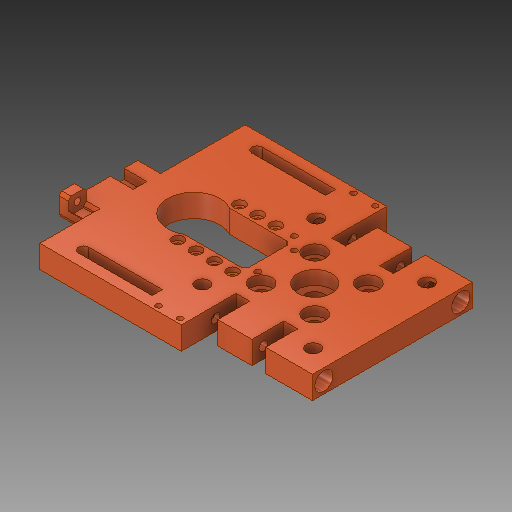
# Autodesk Inventor part: КВ33.044.901 - Щека каретки Z
Saved by Autodesk Inventor 2019 (Build 230136000, 136)
## iProperties
Created: 2019-08-08
Part Number: КВ33.044.901 - Щека каретки Z
Material: Пластик АБС
Document SubType Name: Modeling
Designer: user
Density: 1.06 g/cm^3
Appearance: Гладкий — светло-оранжевый
Mass: 66.4616 g
Surface Area: 302.013 cm^2
Volume: 62.6996 cm^3
Author: user
Autodesk Inventor part; units mm, degrees
(part 1 of 2)
ref_plane "YZ Plane" through (0, 0, 0) normal (1, 0, 0) x (0, 1, 0)
ref_plane "XZ Plane" through (0, 0, 0) normal (0, 1, 0) x (-1, 0, 0)
ref_plane "XY Plane" through (0, 0, 0) normal (0, 0, 1) x (1, 0, 0)
sketch "Эскиз4" plane through (0, 0, 0) normal (0, 1, 0) x (-1, 0, 0)
  circle A0 centre (-24.3, 25) radius 3
  circle A1 centre (24.3, 25) radius 3
  circle A2 centre (24.3, -25) radius 3
  circle A3 centre (-24.3, -25) radius 3
  line L0 (13.5, -21) -> (13.5, -35)
  line L1 (13.5, -35) -> (34, -35)
  line L2 (34, -35) -> (34, 35)
  line L3 (34, 35) -> (13.5, 35)
  line L4 (13.5, 35) -> (13.5, 21)
  line L5 (13.5, 21) -> (7.5, 21)
  line L6 (7.5, 21) -> (7.5, 35)
  line L7 (7.5, 35) -> (-7.5, 35)
  line L8 (-7.5, 35) -> (-7.5, 21)
  line L9 (-7.5, 21) -> (-13.5, 21)
  line L10 (-13.5, 21) -> (-13.5, 35)
  line L11 (-13.5, 35) -> (-34, 35)
  line L12 (-34, 35) -> (-34, -35)
  line L13 (-34, -35) -> (-13.5, -35)
  line L14 (-13.5, -35) -> (-13.5, -21)
  line L15 (-13.5, -21) -> (-7.5, -21)
  line L16 (-7.5, -21) -> (-7.5, -35)
  line L17 (-7.5, -35) -> (7.5, -35)
  line L18 (7.5, -35) -> (7.5, -21)
  line L19 (7.5, -21) -> (13.5, -21)
  circle A4 centre (0, 0) radius 7.5
  circle A5 centre (-11.75, 11.7501) radius 4.65
  circle A6 centre (-11.7501, -11.75) radius 4.65
  line L20 (26, 12) -> (16.3934, 12)
  line L21 (26, -12) -> (26, 12)
  line L22 (16.3933, -12) -> (26, -12)
  arc A7 (16, -9.8634) -> (16.3933, -12) centre (11.75, -11.7501) ccw
  line L23 (16, -9.8634) -> (16, 9.8629)
  arc A8 (16.3934, 12) -> (16, 9.8629) centre (11.7501, 11.75) ccw
  circle A9 centre (-11.75, 11.7501) radius 2.6
  circle A10 centre (-11.7501, -11.75) radius 2.6
  circle A11 centre (11.75, -11.7501) radius 2.6
  circle A12 centre (11.7501, 11.75) radius 2.6
  circle A13 centre (0, 0) radius 4.1
  circle A14 centre (11.7501, 11.75) radius 4.65
  circle A15 centre (11.75, -11.7501) radius 4.65
  constraints: 48 end point, 14 centre point, 4 point on circle, 2 coincident, 6 other
extrude "Выдавливание3" add sketch "Эскиз4" along normal blind 10 contours L19 L18 L17 L16 L15 L14 L13 L12 L11 L10 L9 L8 L7 L6 L5 L4 L3 L2 L1 L0 | A4 | A5 | A6 | L21 L22 A15 L23 A14 L20 | A14 A8 | A7 A15
sketch "Эскиз5" plane through (0, 10, 0) normal (0, 1, 0) x (1, 0, 0)
  circle A0 centre (-24.3, 25) radius 3
  circle A1 centre (24.3, 25) radius 3
  circle A2 centre (24.3, -25) radius 3
  circle A3 centre (-24.3, -25) radius 3
  line L0 (13.5, -21) -> (13.5, -35)
  line L1 (13.5, -35) -> (34, -35)
  line L2 (34, -35) -> (34, 35)
  line L3 (34, 35) -> (13.5, 35)
  line L4 (13.5, 35) -> (13.5, 21)
  line L5 (13.5, 21) -> (7.5, 21)
  line L6 (7.5, 21) -> (7.5, 35)
  line L7 (7.5, 35) -> (-7.5, 35)
  line L8 (-7.5, 35) -> (-7.5, 21)
  line L9 (-7.5, 21) -> (-13.5, 21)
  line L10 (-13.5, 21) -> (-13.5, 35)
  line L11 (-13.5, 35) -> (-34, 35)
  line L12 (-34, 35) -> (-34, -35)
  line L13 (-34, -35) -> (-13.5, -35)
  line L14 (-13.5, -35) -> (-13.5, -21)
  line L15 (-13.5, -21) -> (-7.5, -21)
  line L16 (-7.5, -21) -> (-7.5, -35)
  line L17 (-7.5, -35) -> (7.5, -35)
  line L18 (7.5, -35) -> (7.5, -21)
  line L19 (7.5, -21) -> (13.5, -21)
  circle A4 centre (0, 0) radius 7.5
  circle A5 centre (-11.75, 11.7501) radius 4.65
  circle A6 centre (-11.7501, -11.75) radius 4.65
  line L20 (26, 12) -> (16.3934, 12)
  line L21 (26, -12) -> (26, 12)
  line L22 (16.3933, -12) -> (26, -12)
  arc A7 (16, -9.8634) -> (16.3933, -12) centre (11.75, -11.7501) ccw
  line L23 (16, -9.8634) -> (16, 9.8629)
  arc A8 (16.3934, 12) -> (16, 9.8629) centre (11.7501, 11.75) ccw
  circle A9 centre (-11.75, 11.7501) radius 2.6
  circle A10 centre (-11.7501, -11.75) radius 2.6
  circle A11 centre (11.75, -11.7501) radius 2.6
  circle A12 centre (11.7501, 11.75) radius 2.6
  circle A13 centre (0, 0) radius 4.1
  circle A14 centre (11.75, -11.7501) radius 2.6 projected
  circle A15 centre (11.75, -11.7501) radius 4.65
  circle A16 centre (11.7501, 11.75) radius 4.65
  constraints: 48 end point, 16 centre point, 4 point on circle, 2 coincident, 2 concentric
extrude "Выдавливание4" cut sketch "Эскиз5" against normal blind 4 contours A5 | A6 | A16 A8 | A7 A15
sketch "Эскиз6" plane through (0, 10, 0) normal (0, 1, 0) x (1, 0, 0)
  circle A0 centre (-24.3, 25) radius 3
  circle A1 centre (24.3, 25) radius 3
  circle A2 centre (24.3, -25) radius 3
  circle A3 centre (-24.3, -25) radius 3
  line L0 (13.5, -21) -> (13.5, -35)
  line L1 (13.5, -35) -> (34, -35)
  line L2 (34, -35) -> (34, 35)
  line L3 (34, 35) -> (13.5, 35)
  line L4 (13.5, 35) -> (13.5, 21)
  line L5 (13.5, 21) -> (7.5, 21)
  line L6 (7.5, 21) -> (7.5, 35)
  line L7 (7.5, 35) -> (-7.5, 35)
  line L8 (-7.5, 35) -> (-7.5, 21)
  line L9 (-7.5, 21) -> (-13.5, 21)
  line L10 (-13.5, 21) -> (-13.5, 35)
  line L11 (-13.5, 35) -> (-34, 35)
  line L12 (-34, 35) -> (-34, -35)
  line L13 (-34, -35) -> (-13.5, -35)
  line L14 (-13.5, -35) -> (-13.5, -21)
  line L15 (-13.5, -21) -> (-7.5, -21)
  line L16 (-7.5, -21) -> (-7.5, -35)
  line L17 (-7.5, -35) -> (7.5, -35)
  line L18 (7.5, -35) -> (7.5, -21)
  line L19 (7.5, -21) -> (13.5, -21)
  circle A4 centre (0, 0) radius 7.5
  circle A5 centre (-11.75, 11.7501) radius 4.65
  circle A6 centre (-11.7501, -11.75) radius 4.65
  line L20 (26, 12) -> (16.3934, 12)
  line L21 (26, -12) -> (26, 12)
  line L22 (16.3933, -12) -> (26, -12)
  arc A7 (16, -9.8634) -> (16.3933, -12) centre (11.75, -11.7501) ccw
  line L23 (16, -9.8634) -> (16, 9.8629)
  arc A8 (16.3934, 12) -> (16, 9.8629) centre (11.7501, 11.75) ccw
  circle A9 centre (-11.75, 11.7501) radius 2.6
  circle A10 centre (-11.7501, -11.75) radius 2.6
  circle A11 centre (11.75, -11.7501) radius 2.6
  circle A12 centre (11.7501, 11.75) radius 2.6
  circle A13 centre (0, 0) radius 4.1
  constraints: 48 end point, 14 centre point, 4 point on circle
extrude "Выдавливание5" cut sketch "Эскиз6" against normal blind 6 contours A4
sketch "Эскиз7" plane through (34, 0, 35) normal (1, 0, 0) x (0, 0, -1)
  circle A0 centre (5, 5) radius 2
  circle A1 centre (5, 5) radius 4
  circle A2 centre (65, 5) radius 4
  circle A3 centre (5, 5) radius 4
  line L0 (0, 0) -> (70, 0)
  line L1 (70, 0) -> (70, 10)
  line L2 (0, 10) -> (70, 10)
  line L3 (0, 0) -> (0, 10)
  circle A4 centre (65, 5) radius 2
  circle A5 centre (65, 5) radius 4
  point P0 (35, 0)
  point P1 (35, 0)
  constraints: 8 end point, 6 centre point
extrude "Выдавливание6" cut sketch "Эскиз7" against normal blind 269 contours A0 | A4
sketch "Эскиз8" plane through (34, 0, 35) normal (1, 0, 0) x (0, 0, -1)
  circle A0 centre (5, 5) radius 2
  circle A1 centre (5, 5) radius 4
  circle A2 centre (65, 5) radius 4
  circle A3 centre (5, 5) radius 4
  line L0 (0, 0) -> (70, 0)
  line L1 (70, 0) -> (70, 10)
  line L2 (0, 10) -> (70, 10)
  line L3 (0, 0) -> (0, 10)
  circle A4 centre (65, 5) radius 2
  circle A5 centre (65, 5) radius 4
  point P0 (35, 0)
  point P1 (35, 0)
  constraints: 8 end point, 6 centre point
extrude "Выдавливание7" cut sketch "Эскиз8" against normal blind 15 contours A1 | A2
sketch "Эскиз9" plane through (-34, 0, -35) normal (-1, 0, 0) x (0, 0, 1)
  circle A0 centre (5, 5) radius 2
  circle A1 centre (5, 5) radius 4
  circle A2 centre (65, 5) radius 4
  circle A3 centre (5, 5) radius 4
  line L0 (0, 0) -> (70, 0)
  line L1 (70, 0) -> (70, 10)
  line L2 (0, 10) -> (70, 10)
  line L3 (0, 0) -> (0, 10)
  circle A4 centre (65, 5) radius 2
  circle A5 centre (65, 5) radius 4
  point P0 (35, 0)
  point P1 (35, 0)
  constraints: 8 end point, 6 centre point
extrude "Выдавливание8" cut sketch "Эскиз9" against normal blind 15 contours A1 | A2
sketch "Эскиз17" plane through (-34, 0, -35) normal (-1, 0, 0) x (0, 0, 1)
  line L0 (14, 10) -> (0, 10) projected
  line L1 (70, 0) -> (56, 0) projected
  line L2 (0, 10) -> (70, 10)
  line L3 (70, 10) -> (70, 0)
  line L4 (70, 0) -> (0, 0)
  line L5 (0, 0) -> (0, 10)
  point P0 (35, 0)
  constraints: 8 end point, 2 parallel, 1 horizontal, 1 perpendicular
extrude "Выдавливание14" add sketch "Эскиз17" along normal blind 33
sketch "Эскиз18" plane through (0, 0, 0) normal (0, -1, 0) x (1, 0, 0)
  line L0 (-35.2, -12.6) -> (-35.2, -14.9)
  line L1 (-35.2, -12.6) -> (-33.8, -12.6)
  line L2 (-33.8, -14.9) -> (-33.8, -12.6)
  line L3 (-27.2, -14.9) -> (-33.8, -14.9)
  line L4 (-27.2, -12.6) -> (-27.2, -14.9)
  circle A0 centre (-53, 0) radius 9.15
  circle A1 centre (-53, 0) radius 1.5
  circle A2 centre (-17, 8) radius 1.3
  circle A3 centre (-30.5, 13.5) radius 1.3
  circle A4 centre (-22.5, 13.5) radius 1.3
  circle A5 centre (-38.5, 13.5) radius 1.3
  circle A6 centre (-46.5, 13.5) radius 1.3
  circle A7 centre (-17, -8) radius 1.3
  circle A8 centre (-30.5, -13.5) radius 1.3
  circle A9 centre (-22.5, -13.5) radius 1.3
  circle A10 centre (-38.5, -13.5) radius 1.3
  circle A11 centre (-46.5, -13.5) radius 1.3
  line L5 (-64.0198, -0.1) -> (-63.4796, -0.1)
  line L6 (-64.0198, -7) -> (-64.0198, -0.1)
  arc A12 (-64.0198, -7) -> (-63.9686, -7.75) centre (-58.5, -7) ccw
  line L7 (-61.5, -7.75) -> (-63.9686, -7.75)
  arc A13 (-59.75, -9.5) -> (-61.5, -7.75) centre (-61.5, -9.5) ccw
  line L8 (-59.75, -10) -> (-59.75, -9.5)
  line L9 (-22.1937, -10) -> (-59.75, -10)
  arc A14 (-22.1937, -10) -> (-21.5055, -9.6078) centre (-22.1937, -9.2) ccw
  arc A15 (-21.5055, -9.6078) -> (-20.8922, -8.9945) centre (-20, -10.5) ccw
  arc A16 (-20.8922, -8.9945) -> (-20.5, -8.3063) centre (-21.3, -8.3063) ccw
  line L10 (-20.5, 8.3063) -> (-20.5, -8.3063)
  arc A17 (-20.5, 8.3063) -> (-20.8922, 8.9945) centre (-21.3, 8.3063) ccw
  arc A18 (-21.5055, 9.6078) -> (-20.8922, 8.9945) centre (-20, 10.5) ccw
  arc A19 (-20.8922, 8.9945) -> (-21.5055, 9.6078) centre (-20, 10.5) ccw
  line L11 (-59.75, -11.3229) -> (-59.75, -10)
  arc A20 (-59.75, -11.3229) -> (-58.5, -11.5) centre (-58.4989, -6.9922) ccw
  line L12 (-58.5, -11.5) -> (-51, -11.5)
  line L13 (-51, -12.6) -> (-51, -11.5)
  line L14 (-49.8, -12.6) -> (-51, -12.6)
  line L15 (-49.8, -14.9) -> (-49.8, -12.6)
  line L16 (-43.2, -14.9) -> (-49.8, -14.9)
  line L17 (-43.2, -12.6) -> (-43.2, -14.9)
  line L18 (-41.8, -12.6) -> (-43.2, -12.6)
  line L19 (-41.8, -14.9) -> (-41.8, -12.6)
  line L20 (-35.2, -14.9) -> (-41.8, -14.9)
  line L21 (-35.2, -12.6) -> (-35.2, -14.9)
  line L22 (-33.8, -12.6) -> (-35.2, -12.6)
  line L23 (-33.8, -14.9) -> (-33.8, -12.6)
  line L24 (-27.2, -14.9) -> (-33.8, -14.9)
  line L25 (-27.2, -12.6) -> (-27.2, -14.9)
  line L26 (-25.8, -12.6) -> (-27.2, -12.6)
  line L27 (-25.8, -14.9) -> (-25.8, -12.6)
  line L28 (-19.2, -14.9) -> (-25.8, -14.9)
  line L29 (-19.2, -12.6) -> (-19.2, -14.9)
  line L30 (-17.9802, -12.6) -> (-19.2, -12.6)
  arc A21 (-17.9802, -12.6) -> (-17.9, -12.5198) centre (-19, -11.5) ccw
  line L31 (-17.9, -11.3) -> (-17.9, -12.5198)
  line L32 (-15.6, -11.3) -> (-17.9, -11.3)
  line L33 (-15.6, -4.7) -> (-15.6, -11.3)
  line L34 (-17.9, -4.7) -> (-15.6, -4.7)
  line L35 (-17.9, 4.7) -> (-17.9, -4.7)
  line L36 (-15.6, 4.7) -> (-17.9, 4.7)
  line L37 (-15.6, 11.3) -> (-15.6, 4.7)
  line L38 (-17.9, 11.3) -> (-15.6, 11.3)
  line L39 (-17.9, 12.5198) -> (-17.9, 11.3)
  arc A22 (-17.9, 12.5198) -> (-17.9802, 12.6) centre (-19, 11.5) ccw
  line L40 (-19.2, 12.6) -> (-17.9802, 12.6)
  line L41 (-19.2, 14.9) -> (-19.2, 12.6)
  line L42 (-25.8, 14.9) -> (-19.2, 14.9)
  line L43 (-25.8, 12.6) -> (-25.8, 14.9)
  line L44 (-27.2, 12.6) -> (-25.8, 12.6)
  line L45 (-27.2, 14.9) -> (-27.2, 12.6)
  line L46 (-33.8, 14.9) -> (-27.2, 14.9)
  line L47 (-33.8, 12.6) -> (-33.8, 14.9)
  line L48 (-35.2, 12.6) -> (-33.8, 12.6)
  line L49 (-35.2, 14.9) -> (-35.2, 12.6)
  line L50 (-41.8, 14.9) -> (-35.2, 14.9)
  line L51 (-41.8, 12.6) -> (-41.8, 14.9)
  line L52 (-43.2, 12.6) -> (-41.8, 12.6)
  line L53 (-43.2, 14.9) -> (-43.2, 12.6)
  line L54 (-49.8, 14.9) -> (-43.2, 14.9)
  line L55 (-49.8, 12.6) -> (-49.8, 14.9)
  line L56 (-51, 12.6) -> (-49.8, 12.6)
  line L57 (-51, 11.5) -> (-51, 12.6)
  line L58 (-58.5, 11.5) -> (-51, 11.5)
  arc A23 (-58.5, 11.5) -> (-59.75, 11.3229) centre (-58.4989, 6.9922) ccw
  line L59 (-59.75, 10) -> (-59.75, 11.3229)
  line L60 (-59.75, 9.5) -> (-59.75, 10)
  arc A24 (-61.5, 7.75) -> (-59.75, 9.5) centre (-61.5, 9.5) ccw
  line L61 (-63.9686, 7.75) -> (-61.5, 7.75)
  arc A25 (-63.9686, 7.75) -> (-64.0198, 7) centre (-58.5, 7) ccw
  line L62 (-64.0198, 0.1) -> (-64.0198, 7)
  line L63 (-63.4796, 0.1) -> (-64.0198, 0.1)
  arc A26 (-20.8922, -8.9945) -> (-21.5055, -9.6078) centre (-20, -10.5) ccw
  arc A27 (-21.5055, 9.6078) -> (-22.1937, 10) centre (-22.1937, 9.2) ccw
  line L64 (-59.75, 10) -> (-22.1937, 10)
  line L65 (0, 0) -> (-34, 0)
  line L66 (-34, 0) -> (-53, 0)
  line L67 (-53, -9.15) -> (-53, -10)
  line L68 (-53, 10) -> (-53, 9.15)
  dimension "d62" = 34
  dimension "d63" = 19
  constraints: 138 end point, 34 point on circle, 28 centre point, 4 point on line, 2 horizontal, 1 perpendicular
  measures "d62" distance of L65.start L65.end
  measures "d63" distance of L65.end L66.end
extrude "Выдавливание15" cut sketch "Эскиз18" against normal blind 23 contours L67 A0 L66 L65 L10 A16 A26 A14 L9 | A0 | L68 L64 A27 A18 A17 L10 L65 L66 A0 | A1 | A2 | A3 | A4 | A5 | A6 | A7 | A8 | A9 | A10 | A11
sketch "Эскиз19" plane through (0, 0, 0) normal (0, -1, 0) x (1, 0, 0)
  arc A0 (-53, 9.15) -> (-53, -9.15) centre (-53, 0) ccw projected
  circle A1 centre (-53, 0) radius 11.5
  point P0 (0, 0)
  dimension "d66" = 23
  constraints: 1 centre point, 1 coincident
  measures "d66" diameter of A1
extrude "Выдавливание16" cut sketch "Эскиз19" against normal blind 23
sketch "Эскиз20" plane through (0, 10, 0) normal (0, 1, 0) x (1, 0, 0)
  circle A0 centre (-22.5, -13.5) radius 1.3 projected
  circle A1 centre (-22.5, -13.5) radius 2.5
  circle A2 centre (-30.5, -13.5) radius 1.3 projected
  circle A3 centre (-30.5, -13.5) radius 2.5
  circle A4 centre (-38.5, -13.5) radius 1.3 projected
  circle A5 centre (-38.5, -13.5) radius 2.5
  circle A6 centre (-46.5, -13.5) radius 1.3 projected
  circle A7 centre (-46.5, -13.5) radius 2.5
  circle A8 centre (-46.5, 13.5) radius 1.3 projected
  circle A9 centre (-46.5, 13.5) radius 2.5
  circle A10 centre (-38.5, 13.5) radius 1.3 projected
  circle A11 centre (-38.5, 13.5) radius 2.5
  circle A12 centre (-30.5, 13.5) radius 1.3 projected
  circle A13 centre (-30.5, 13.5) radius 2.5
  circle A14 centre (-22.5, 13.5) radius 1.3 projected
  circle A15 centre (-22.5, 13.5) radius 2.5
  point P0 (0, 0)
  dimension "d69" = 5
  dimension "d70" = 5
  dimension "d71" = 5
  dimension "d72" = 5
  dimension "d73" = 5
  dimension "d74" = 5
  dimension "d75" = 5
  dimension "d76" = 5
  constraints: 8 centre point, 8 coincident
  measures "d69" diameter of A1
  measures "d70" diameter of A3
  measures "d71" diameter of A5
  measures "d72" diameter of A7
  measures "d73" diameter of A9
  measures "d74" diameter of A11
  measures "d75" diameter of A13
  measures "d76" diameter of A15
extrude "Выдавливание17" cut sketch "Эскиз20" against normal blind 2 contours A0 | A1 | A2 | A3 | A4 | A5 | A6 | A7 | A8 | A9 | A10 | A11 | A12 | A13 | A14
move faces "Перенос3" translate (0, 0, -10) faces at (-49.1667, 6.6667, -35)
move faces "Перенос4" translate (0, 0, 10) faces at (-31.3333, 6.6667, 35)
sketch "Эскиз21" plane through (0, 10, 0) normal (0, 1, 0) x (1, 0, 0)
  line L0 (-13.5, -45) -> (-67, -45) projected
  line L1 (-40.25, -45) -> (-40.25, -38)
  line L2 (-13.5, 45) -> (-67, 45) projected
  line L3 (-40.25, 45) -> (-40.25, 38)
  line L4 (-17.1684, -38) -> (-63.3316, -38) construction
  line L5 (-17.1684, -35.75) -> (-63.3316, -35.75)
  line L6 (-63.3316, -40.25) -> (-17.1684, -40.25)
  arc A0 (-17.1684, -40.25) -> (-17.1684, -35.75) centre (-17.1684, -38) ccw
  arc A1 (-63.3316, -35.75) -> (-63.3316, -40.25) centre (-63.3316, -38) ccw
  line L7 (-17.1684, 38) -> (-63.3316, 38) construction
  line L8 (-17.1684, 40.25) -> (-63.3316, 40.25)
  line L9 (-63.3316, 35.75) -> (-17.1684, 35.75)
  arc A2 (-17.1684, 35.75) -> (-17.1684, 40.25) centre (-17.1684, 38) ccw
  arc A3 (-63.3316, 40.25) -> (-63.3316, 35.75) centre (-63.3316, 38) ccw
  point P0 (0, 0)
  dimension "d85" = 7
  dimension "d86" = 7
  dimension "d87" = 90
  dimension "d88" = 4.5
  dimension "d89" = 4.5
  constraints: 20 end point, 8 point on circle, 8 tangent, 4 centre point, 4 midpoint, 2 horizontal, 2 parallel, 1 vertical
  measures "d85" distance of L1.start L1.end
  measures "d86" distance of L3.start L3.end
  measures "d87" angle of L2 L3
  measures "d88" diameter of A1
  measures "d89" diameter of A3
extrude "Выдавливание18" cut sketch "Эскиз21" against normal blind 15.5
move faces "Перенос5" translate (-8.5, 0, 0) faces at (-67, 3.3333, 15)
sketch "Эскиз24" plane through (-75.5, 0, -45) normal (-1, 0, 0) x (0, 0, 1)
  line L0 (90, 0) -> (90, 10) projected
  line L1 (90, 0) -> (66, 0) projected
  line L2 (90, 0) -> (90, 5.8)
  line L3 (90, 5.8) -> (49.1, 5.8)
  line L4 (49.1, 5.8) -> (90, 5.8)
  line L5 (90, 5.8) -> (90, 10)
  line L6 (90, 10) -> (49.1, 10)
  line L7 (49.1, 10) -> (49.1, 5.8)
  line L8 (49.1, 10) -> (71.6, 10)
  line L9 (90, 10) -> (0, 10) projected
  line L10 (71.6, 10) -> (71.6, 5.8)
  point P0 (45, 0)
  dimension "d103" = 5.8
  dimension "d104" = 40.9
  dimension "d105" = 22.5
  constraints: 16 end point, 3 perpendicular, 3 point on line, 2 parallel, 1 horizontal
  measures "d103" distance of L0.start L2.end
  measures "d104" distance of L2.end L3.end
  measures "d105" distance of L6.end L8.end
extrude "Выдавливание20" add sketch "Эскиз24" along normal blind 10 contours L3 L7 L6 L10
sketch "Эскиз25" plane through (-75.5, 0, -45) normal (-1, 0, 0) x (0, 0, 1)
  line L0 (49.1, 5.8) -> (49.1, 10) projected
  line L1 (49.1, 5.8) -> (43.1, 5.8)
  line L2 (43.1, 5.8) -> (43.1, 0)
  line L3 (43.1, 0) -> (49.1, 0)
  line L4 (49.1, 0) -> (49.1, 5.8)
  line L5 (43.1, 5.8) -> (37.1, 5.8)
  line L6 (37.1, 5.8) -> (37.1, 10)
  line L7 (37.1, 10) -> (43.1, 10)
  line L8 (43.1, 10) -> (43.1, 5.8)
  line L9 (41.9955, 5.8) -> (43.1, 4.6332)
  line L10 (49.1, 4.6332) -> (50.3326, 5.8)
  line L11 (71.6, 5.8) -> (49.1, 5.8) projected
  line L12 (49.1, 5.8) -> (50.3326, 5.8)
  point P0 (45, 0)
  dimension "d108" = 6
  dimension "d109" = 5.8
  dimension "d110" = 6
  dimension "d111" = 4.2
  constraints: 22 end point, 4 parallel, 4 point on line, 3 horizontal, 3 perpendicular
  measures "d108" distance of L3.end L2.end
  measures "d109" distance of L2.end L1.end
  measures "d110" distance of L6.end L7.end
  measures "d111" distance of L5.end L6.end
extrude "Выдавливание21" add sketch "Эскиз25" along normal blind 10
sketch "Эскиз26" plane through (-85.5, 0, -45) normal (-1, 0, 0) x (0, 0, 1)
  line L0 (71.6, 5.8) -> (71.6, 10) projected
  line L1 (71.6, 7.9) -> (67.5, 7.9)
  line L2 (71.6, 5.8) -> (63.6, 5.8)
  line L3 (63.6, 5.8) -> (63.6, 15.1)
  line L4 (63.6, 15.1) -> (71.6, 15.1)
  line L5 (71.6, 15.1) -> (71.6, 5.8)
  line L6 (67.5, 7.9) -> (67.5, 11.7)
  circle A0 centre (67.5, 11.7) radius 1.5
  point P0 (45, 0)
  dimension "d114" = 4.1
  dimension "d115" = 8
  dimension "d116" = 9.3
  dimension "d117" = 3.8
  dimension "d118" = 3
  constraints: 12 end point, 2 horizontal, 2 parallel, 1 centre point, 1 coincident, 1 midpoint, 1 perpendicular, 1 vertical
  measures "d114" distance of L1.start L1.end
  measures "d115" distance of L3.end L4.end
  measures "d116" distance of L2.end L3.end
  measures "d117" distance of L1.end L6.end
  measures "d118" diameter of A0
extrude "Выдавливание22" add sketch "Эскиз26" against normal blind 4
sketch "Эскиз29" plane through (0, 10, 0) normal (0, 1, 0) x (1, 0, 0)
  line L0 (-81.5, -21) -> (-81.5, -24) projected
  line L1 (-81.5, -21) -> (-81.5, -20)
  line L2 (-81.5, -18.6) -> (-81.5, -26.6) projected
  line L3 (-75.5, -26.6) -> (-75.5, -5.3326) projected
  line L4 (-81.5, -20) -> (-75.5, -20)
  line L5 (-75.5, -20) -> (-75.5, -25)
  line L6 (-75.5, -25) -> (-81.5, -25)
  line L7 (-81.5, -25) -> (-81.5, -20)
  point P0 (0, 0)
  dimension "d127" = 1
  dimension "d128" = 5
  constraints: 10 end point, 2 parallel, 2 point on line, 1 horizontal, 1 perpendicular
  measures "d127" distance of L0.start L1.end
  measures "d128" distance of L4.end L5.end
extrude "Выдавливание25" cut sketch "Эскиз29" against normal blind 2
chamfer "Фаска2" distance 1.25 angle 45 2 edges at (-78.5, 10, 20) (-78.5, 10, 25)
chamfer "Фаска3" distance 1.25 angle 45 2 edges at (-83.5, 15.1, 26.6) (-83.5, 15.1, 18.6)
sketch "Эскиз30" plane through (-75.5, 0, 45) normal (-1, 0, 0) x (0, 0, 1)
  circle A0 centre (-15, 5) radius 2 projected
  circle A1 centre (-15, 5) radius 4
  circle A2 centre (-75, 5) radius 2 projected
  circle A3 centre (-75, 5) radius 4
  point P0 (-45, 0)
  constraints: 2 centre point, 2 coincident
extrude "Выдавливание26" cut sketch "Эскиз30" against normal blind 56.25 and the other way blind 12.125 contours A0 | A1 | A2 | A3
sketch "Эскиз32" plane through (0, 0, 0) normal (0, -1, 0) x (1, 0, 0)
  line L0 (-13.5, -21) -> (-13.5, -45) projected
  line L1 (-13.5, -45) -> (-31.0536, -45)
  line L2 (-31.0536, -45) -> (-31.0536, -35.2417)
  line L3 (-31.0536, -35.2417) -> (-13.5, -35.2417)
  line L4 (-13.5, -35.2417) -> (-13.5, -45)
  line L5 (-13.5, 45) -> (-31.0536, 45)
  line L6 (-31.0536, 45) -> (-31.0536, 35)
  line L7 (-31.0536, 35) -> (-13.5, 35)
  line L8 (-13.5, 35) -> (-13.5, 45)
  point P0 (0, 0)
  dimension "d145" = 10
  constraints: 16 end point, 4 parallel, 2 horizontal, 2 perpendicular, 1 point on line
  measures "d145" distance of L7.end L5.start
extrude "Выдавливание27" add sketch "Эскиз32" against normal blind 10
sketch "Эскиз31" plane through (0, 0, 0) normal (0, -1, 0) x (1, 0, 0)
  line L0 (-11.163, 50.525) -> (-11.6756, 50.525)
  line L1 (-11.6756, 50.525) -> (-11.7673, 49.091)
  arc A0 (-15.9587, 49.091) -> (-11.7673, 49.091) centre (-13.863, 49.225) ccw
  line L2 (-15.9587, 49.091) -> (-16.0504, 50.525)
  line L3 (-16.0504, 50.525) -> (-20.3387, 50.525)
  arc A1 (-20.3387, 50.525) -> (-20.4094, 50.4957) centre (-20.3387, 50.425) ccw
  line L4 (-20.4094, 50.4957) -> (-20.7337, 50.1714)
  arc A2 (-21.0872, 50.025) -> (-20.7337, 50.1714) centre (-21.0872, 50.525) ccw
  line L5 (-21.0872, 50.025) -> (-30.763, 50.025)
  arc A3 (-30.763, 50.025) -> (-30.863, 49.925) centre (-30.763, 49.925) ccw
  line L6 (-30.863, 49.925) -> (-30.863, 40.775)
  arc A4 (-30.863, 40.775) -> (-30.763, 40.675) centre (-30.763, 40.775) ccw
  line L7 (-30.763, 40.675) -> (-27.8372, 40.675)
  arc A5 (-27.4837, 40.5285) -> (-27.8372, 40.675) centre (-27.8372, 40.175) ccw
  line L8 (-27.4837, 40.5285) -> (-27.1594, 40.2043)
  arc A6 (-27.1594, 40.2043) -> (-27.0887, 40.175) centre (-27.0887, 40.275) ccw
  line L9 (-27.0887, 40.175) -> (-24.3372, 40.175)
  arc A7 (-24.3372, 40.175) -> (-24.2665, 40.2043) centre (-24.3372, 40.275) ccw
  line L10 (-24.2665, 40.2043) -> (-23.9423, 40.5285)
  arc A8 (-23.5887, 40.675) -> (-23.9423, 40.5285) centre (-23.5887, 40.175) ccw
  line L11 (-23.5887, 40.675) -> (-18.3372, 40.675)
  arc A9 (-17.9837, 40.5285) -> (-18.3372, 40.675) centre (-18.3372, 40.175) ccw
  line L12 (-17.9837, 40.5285) -> (-17.6594, 40.2043)
  arc A10 (-17.6594, 40.2043) -> (-17.5887, 40.175) centre (-17.5887, 40.275) ccw
  line L13 (-17.5887, 40.175) -> (-14.8372, 40.175)
  arc A11 (-14.8372, 40.175) -> (-14.7665, 40.2043) centre (-14.8372, 40.275) ccw
  line L14 (-14.7665, 40.2043) -> (-14.4423, 40.5285)
  arc A12 (-14.0887, 40.675) -> (-14.4423, 40.5285) centre (-14.0887, 40.175) ccw
  line L15 (-14.0887, 40.675) -> (-11.163, 40.675)
  arc A13 (-11.163, 40.675) -> (-11.063, 40.775) centre (-11.163, 40.775) ccw
  line L16 (-11.063, 40.775) -> (-11.063, 50.425)
  arc A14 (-11.063, 50.425) -> (-11.163, 50.525) centre (-11.163, 50.425) ccw
  circle A15 centre (-16.213, 42.725) radius 1.25
  circle A16 centre (-25.713, 42.725) radius 1.25
  line L17 (-26.8863, 44.975) -> (-26.2696, 46.275)
  line L18 (-26.2696, 46.275) -> (-26.253, 46.275)
  line L19 (-26.253, 46.275) -> (-25.653, 44.975)
  line L20 (-25.653, 44.975) -> (-25.7798, 44.975)
  line L21 (-25.7798, 44.975) -> (-25.972, 45.3916)
  line L22 (-25.972, 45.3916) -> (-26.5613, 45.3916)
  line L23 (-26.5613, 45.3916) -> (-26.759, 44.975)
  line L24 (-26.759, 44.975) -> (-26.8863, 44.975)
  spline S0 degree 3 poles (-24.0663, 45.9114) (-24.0665, 45.9203) (-24.067, 45.9378) (-24.0711, 45.9634) (-24.0773, 45.9881) (-24.0862, 46.012) (-24.098, 46.0348) (-24.1122, 46.0566) (-24.1287, 46.0777) (-24.1478, 46.0974) (-24.1688, 46.1155) (-24.1909, 46.1315) (-24.2143, 46.1449) (-24.2389, 46.1559) (-24.2646, 46.1645) (-24.2915, 46.1705) (-24.3195, 46.1742) (-24.3386, 46.1747) (-24.3483, 46.175) knots 0 0 0 0 0.061965 0.122122 0.180988 0.239933 0.299906 0.359989 0.421776 0.486576 0.551535 0.615018 0.677259 0.73973 0.80305 0.866495 0.931973 1 1 1 1
  spline S1 degree 3 poles (-24.3483, 46.175) (-24.3585, 46.1747) (-24.3785, 46.1742) (-24.4078, 46.1705) (-24.4357, 46.1642) (-24.4624, 46.1556) (-24.4879, 46.1447) (-24.512, 46.1311) (-24.5347, 46.1148) (-24.556, 46.0964) (-24.5756, 46.0758) (-24.5929, 46.0529) (-24.6079, 46.0281) (-24.6211, 46.0014) (-24.6318, 45.9726) (-24.6399, 45.9418) (-24.6464, 45.9091) (-24.6485, 45.8865) (-24.6496, 45.875) knots 0 0 0 0 0.064439 0.126547 0.186887 0.245878 0.304041 0.362191 0.420976 0.48066 0.5406 0.600689 0.661936 0.724443 0.789038 0.856314 0.926352 1 1 1 1
  line L25 (-24.6496, 45.875) -> (-24.7663, 45.875)
  spline S2 degree 3 poles (-24.7663, 45.875) (-24.7655, 45.8904) (-24.7641, 45.9208) (-24.7571, 45.9652) (-24.7471, 46.0075) (-24.7329, 46.0476) (-24.7153, 46.0857) (-24.6943, 46.1217) (-24.6693, 46.1555) (-24.641, 46.1868) (-24.6103, 46.2155) (-24.5771, 46.2402) (-24.5422, 46.2611) (-24.5058, 46.2786) (-24.4674, 46.2917) (-24.4273, 46.3015) (-24.3854, 46.3073) (-24.3569, 46.308) (-24.3423, 46.3083) knots 0 0 0 0 0.068791 0.135103 0.198979 0.261904 0.323495 0.385195 0.446969 0.509765 0.572251 0.633405 0.693251 0.752583 0.812579 0.873275 0.93555 1 1 1 1
  spline S3 degree 3 poles (-24.3423, 46.3083) (-24.3281, 46.308) (-24.3001, 46.3073) (-24.2592, 46.3017) (-24.2203, 46.2929) (-24.1834, 46.2805) (-24.1489, 46.2638) (-24.1164, 46.2439) (-24.0856, 46.2208) (-24.0579, 46.1935) (-24.0325, 46.1645) (-24.0105, 46.1335) (-23.9917, 46.1015) (-23.976, 46.0682) (-23.9645, 46.0333) (-23.9557, 45.9974) (-23.9508, 45.96) (-23.95, 45.9347) (-23.9496, 45.9218) knots 0 0 0 0 0.069475 0.136517 0.200789 0.26383 0.325735 0.387291 0.449509 0.512968 0.576275 0.63758 0.697903 0.757172 0.816599 0.876653 0.93729 1 1 1 1
  spline S4 degree 3 poles (-23.9496, 45.9218) (-23.9503, 45.9037) (-23.9515, 45.8678) (-23.9622, 45.8151) (-23.9788, 45.764) (-23.9989, 45.7229) (-24.0191, 45.6897) (-24.0374, 45.6624) (-24.0587, 45.633) (-24.0835, 45.6017) (-24.1111, 45.568) (-24.142, 45.5322) (-24.1762, 45.4945) (-24.2002, 45.4688) (-24.2127, 45.4554) knots 0 0 0 0 0.098702 0.195672 0.292422 0.391343 0.444462 0.504229 0.570352 0.642546 0.722288 0.807921 0.90047 1 1 1 1
  line L26 (-24.2127, 45.4554) -> (-24.5379, 45.1083)
  line L27 (-24.5379, 45.1083) -> (-23.933, 45.1083)
  line L28 (-23.933, 45.1083) -> (-23.933, 44.975)
  line L29 (-23.933, 44.975) -> (-24.8163, 44.975)
  line L30 (-24.8163, 44.975) -> (-24.3121, 45.513)
  spline S5 degree 3 poles (-24.3121, 45.513) (-24.2999, 45.5258) (-24.2763, 45.5504) (-24.2429, 45.5863) (-24.213, 45.6197) (-24.1862, 45.6504) (-24.1633, 45.6788) (-24.1429, 45.7041) (-24.1266, 45.7275) (-24.1088, 45.7545) (-24.0917, 45.7875) (-24.0769, 45.8278) (-24.0679, 45.8693) (-24.0669, 45.8973) (-24.0663, 45.9114) knots 0 0 0 0 0.110803 0.212829 0.306101 0.390647 0.466924 0.534481 0.593587 0.644557 0.7362 0.825024 0.911986 1 1 1 1
  line L31 (-23.5563, 45.625) -> (-23.423, 46.275)
  line L32 (-23.423, 46.275) -> (-22.8896, 46.275)
  line L33 (-22.8896, 46.275) -> (-22.8896, 46.1416)
  line L34 (-22.8896, 46.1416) -> (-23.3318, 46.1416)
  line L35 (-23.3318, 46.1416) -> (-23.4019, 45.7997)
  spline S6 degree 3 poles (-23.4019, 45.7997) (-23.3881, 45.8035) (-23.3615, 45.8109) (-23.3221, 45.819) (-23.2847, 45.824) (-23.2605, 45.8246) (-23.2488, 45.825) knots 0 0 0 0 0.275068 0.532901 0.773973 1 1 1 1
  spline S7 degree 3 poles (-23.2488, 45.825) (-23.2342, 45.8247) (-23.2057, 45.824) (-23.1639, 45.8181) (-23.1241, 45.8088) (-23.0862, 45.7957) (-23.0502, 45.779) (-23.0165, 45.7582) (-22.9845, 45.7339) (-22.9548, 45.7059) (-22.9278, 45.6751) (-22.9041, 45.642) (-22.884, 45.6068) (-22.8679, 45.5694) (-22.8549, 45.5301) (-22.8463, 45.4884) (-22.8406, 45.4447) (-22.84, 45.4149) (-22.8396, 45.3997) knots 0 0 0 0 0.065808 0.129394 0.190894 0.251281 0.310815 0.370371 0.430768 0.492881 0.555104 0.616067 0.677256 0.73826 0.800762 0.864778 0.931045 1 1 1 1
  spline S8 degree 3 poles (-22.8396, 45.3997) (-22.8399, 45.3891) (-22.8404, 45.3681) (-22.8429, 45.3368) (-22.8477, 45.3062) (-22.8541, 45.2763) (-22.8625, 45.2471) (-22.8726, 45.2185) (-22.885, 45.1907) (-22.8986, 45.1635) (-22.914, 45.1374) (-22.931, 45.113) (-22.9489, 45.0899) (-22.9683, 45.0685) (-22.9891, 45.0487) (-23.0113, 45.0305) (-23.0346, 45.0136) (-23.0593, 44.9987) (-23.085, 44.985) (-23.112, 44.9737) (-23.1397, 44.9636) (-23.1684, 44.9556) (-23.1981, 44.9493) (-23.229, 44.945) (-23.2607, 44.9419) (-23.2822, 44.9417) (-23.293, 44.9416) knots 0 0 0 0 0.044014 0.087434 0.130118 0.172554 0.214555 0.256298 0.298438 0.340849 0.382715 0.423924 0.464246 0.504074 0.543862 0.583567 0.623094 0.663229 0.703551 0.743938 0.784541 0.82575 0.867757 0.910745 0.954914 1 1 1 1
  spline S9 degree 3 poles (-23.293, 44.9416) (-23.306, 44.9419) (-23.3315, 44.9424) (-23.3688, 44.9477) (-23.4047, 44.9552) (-23.4389, 44.9666) (-23.4718, 44.9809) (-23.5028, 44.9989) (-23.5327, 45.0193) (-23.5604, 45.0434) (-23.5861, 45.0698) (-23.609, 45.0983) (-23.6295, 45.1287) (-23.6472, 45.161) (-23.6622, 45.1951) (-23.674, 45.2312) (-23.6836, 45.269) (-23.6876, 45.2951) (-23.6896, 45.3083) knots 0 0 0 0 0.065421 0.128708 0.190236 0.250724 0.310637 0.370766 0.431615 0.493523 0.555883 0.617342 0.678668 0.740711 0.802985 0.866803 0.932347 1 1 1 1
  line L36 (-23.6896, 45.3083) -> (-23.573, 45.3083)
  spline S10 degree 3 poles (-23.573, 45.3083) (-23.5701, 45.2959) (-23.5646, 45.2721) (-23.5525, 45.2386) (-23.5377, 45.2088) (-23.5201, 45.1822) (-23.4991, 45.159) (-23.4751, 45.1383) (-23.4482, 45.1197) (-23.4184, 45.1042) (-23.3869, 45.0909) (-23.3539, 45.0821) (-23.3203, 45.0759) (-23.2977, 45.0753) (-23.2863, 45.075) knots 0 0 0 0 0.094687 0.181994 0.264377 0.34218 0.418618 0.496509 0.577369 0.661511 0.746733 0.831258 0.915206 1 1 1 1
  spline S11 degree 3 poles (-23.2863, 45.075) (-23.2751, 45.0753) (-23.2532, 45.0759) (-23.221, 45.0805) (-23.1898, 45.0876) (-23.1601, 45.0983) (-23.1313, 45.1112) (-23.1041, 45.1278) (-23.0778, 45.1469) (-23.0531, 45.1688) (-23.0305, 45.1929) (-23.0106, 45.2188) (-22.9939, 45.2463) (-22.9799, 45.2751) (-22.9693, 45.3054) (-22.9617, 45.3372) (-22.9572, 45.3704) (-22.9566, 45.3931) (-22.9563, 45.4047) knots 0 0 0 0 0.064207 0.126425 0.18768 0.248216 0.308305 0.369661 0.431699 0.495947 0.559758 0.622295 0.683911 0.745092 0.80674 0.869087 0.93329 1 1 1 1
  spline S12 degree 3 poles (-22.9563, 45.4047) (-22.9566, 45.4151) (-22.957, 45.4355) (-22.9609, 45.4654) (-22.9677, 45.4936) (-22.9772, 45.5204) (-22.9892, 45.5457) (-23.0038, 45.5697) (-23.0214, 45.5918) (-23.0415, 45.6123) (-23.0635, 45.6312) (-23.0878, 45.6473) (-23.1139, 45.6608) (-23.1415, 45.6725) (-23.1712, 45.6809) (-23.2024, 45.6872) (-23.2356, 45.6909) (-23.2582, 45.6914) (-23.2698, 45.6916) knots 0 0 0 0 0.065351 0.127916 0.18836 0.247216 0.30563 0.36377 0.422661 0.482687 0.5433 0.604118 0.664965 0.727413 0.791468 0.858055 0.927037 1 1 1 1
  spline S13 degree 3 poles (-23.2698, 45.6916) (-23.2799, 45.6914) (-23.3007, 45.691) (-23.3326, 45.6877) (-23.3662, 45.6824) (-23.4012, 45.6751) (-23.4378, 45.6656) (-23.476, 45.6542) (-23.5158, 45.6406) (-23.5425, 45.6303) (-23.5563, 45.625) knots 0 0 0 0 0.102203 0.211023 0.3251 0.446502 0.573788 0.708901 0.850358 1 1 1 1
  line L37 (-20.1096, 44.975) -> (-19.493, 46.275)
  line L38 (-19.493, 46.275) -> (-19.4763, 46.275)
  line L39 (-19.4763, 46.275) -> (-18.8763, 44.975)
  line L40 (-18.8763, 44.975) -> (-19.0031, 44.975)
  line L41 (-19.0031, 44.975) -> (-19.1953, 45.3916)
  line L42 (-19.1953, 45.3916) -> (-19.7846, 45.3916)
  line L43 (-19.7846, 45.3916) -> (-19.9823, 44.975)
  line L44 (-19.9823, 44.975) -> (-20.1096, 44.975)
  spline S14 degree 3 poles (-18.5996, 45.6325) (-18.5991, 45.6559) (-18.5979, 45.7019) (-18.5883, 45.7694) (-18.5727, 45.8341) (-18.5507, 45.8958) (-18.5227, 45.9549) (-18.4882, 46.011) (-18.4474, 46.0643) (-18.4008, 46.1141) (-18.3497, 46.1596) (-18.295, 46.1996) (-18.2368, 46.2329) (-18.1757, 46.2608) (-18.1112, 46.2822) (-18.0436, 46.2972) (-17.9729, 46.3065) (-17.9247, 46.3077) (-17.9002, 46.3083) knots 0 0 0 0 0.064558 0.127014 0.187955 0.248014 0.307748 0.368235 0.42947 0.492743 0.556258 0.618217 0.679655 0.741246 0.803415 0.866815 0.932328 1 1 1 1
  spline S15 degree 3 poles (-17.9002, 46.3083) (-17.8852, 46.3081) (-17.8557, 46.3078) (-17.8119, 46.3043) (-17.7693, 46.2985) (-17.7279, 46.2907) (-17.6874, 46.281) (-17.6481, 46.2683) (-17.6098, 46.2538) (-17.5727, 46.2371) (-17.5371, 46.2183) (-17.5029, 46.1978) (-17.4704, 46.1754) (-17.4394, 46.1513) (-17.4104, 46.1252) (-17.3825, 46.0976) (-17.3568, 46.0679) (-17.3409, 46.0469) (-17.333, 46.0364) knots 0 0 0 0 0.068548 0.135683 0.201215 0.265682 0.329267 0.392395 0.45507 0.517127 0.57879 0.63974 0.700192 0.759806 0.819628 0.879355 0.939512 1 1 1 1
  line L45 (-17.333, 46.0364) -> (-17.4351, 45.9583)
  spline S16 degree 3 poles (-17.4351, 45.9583) (-17.4423, 45.967) (-17.4568, 45.9842) (-17.4801, 46.0084) (-17.5043, 46.0311) (-17.5296, 46.0524) (-17.5562, 46.0715) (-17.5836, 46.0894) (-17.6123, 46.1055) (-17.652, 46.125) (-17.7038, 46.1453) (-17.7691, 46.1623) (-17.8373, 46.1732) (-17.8838, 46.1744) (-17.9075, 46.175) knots 0 0 0 0 0.063163 0.125475 0.187121 0.248294 0.309295 0.36985 0.430973 0.492456 0.616148 0.740844 0.868183 1 1 1 1
  spline S17 degree 3 poles (-17.9075, 46.175) (-17.9205, 46.1748) (-17.9464, 46.1745) (-17.9849, 46.1706) (-18.0227, 46.165) (-18.0597, 46.1568) (-18.096, 46.1464) (-18.1317, 46.134) (-18.1663, 46.1187) (-18.2003, 46.1017) (-18.2329, 46.0825) (-18.2638, 46.0616) (-18.2928, 46.0392) (-18.3199, 46.0151) (-18.3452, 45.9897) (-18.3685, 45.9624) (-18.3898, 45.9335) (-18.4094, 45.9033) (-18.4269, 45.8719) (-18.4416, 45.8392) (-18.4546, 45.8057) (-18.4649, 45.7711) (-18.473, 45.7356) (-18.4786, 45.6991) (-18.4825, 45.6618) (-18.4828, 45.6364) (-18.483, 45.6237) knots 0 0 0 0 0.043955 0.087502 0.130463 0.172752 0.215403 0.25765 0.300153 0.343121 0.385925 0.427686 0.468818 0.509492 0.549883 0.58998 0.630405 0.670869 0.711384 0.751627 0.791776 0.832459 0.873319 0.914543 0.956924 1 1 1 1
  spline S18 degree 3 poles (-18.483, 45.6237) (-18.4825, 45.6044) (-18.4816, 45.5667) (-18.4734, 45.5115) (-18.461, 45.4585) (-18.4423, 45.4082) (-18.4193, 45.36) (-18.3902, 45.3146) (-18.3566, 45.2714) (-18.3179, 45.2313) (-18.2754, 45.1947) (-18.2298, 45.1625) (-18.1812, 45.1356) (-18.1302, 45.1133) (-18.0763, 45.0961) (-18.0197, 45.084) (-17.9605, 45.0761) (-17.92, 45.0753) (-17.8994, 45.075) knots 0 0 0 0 0.064323 0.12629 0.186726 0.246146 0.305576 0.365429 0.426326 0.48884 0.551725 0.613919 0.675484 0.737334 0.800229 0.864502 0.931041 1 1 1 1
  spline S19 degree 3 poles (-17.8994, 45.075) (-17.8767, 45.0756) (-17.832, 45.0768) (-17.7665, 45.0873) (-17.7038, 45.1042) (-17.6439, 45.128) (-17.5869, 45.1588) (-17.5328, 45.1962) (-17.4816, 45.2405) (-17.4508, 45.2744) (-17.4351, 45.2916) knots 0 0 0 0 0.128515 0.252949 0.374755 0.49594 0.617181 0.740909 0.867811 1 1 1 1
  line L46 (-17.4351, 45.2916) -> (-17.333, 45.2143)
  spline S20 degree 3 poles (-17.333, 45.2143) (-17.3412, 45.2037) (-17.3576, 45.1825) (-17.3841, 45.1527) (-17.4121, 45.1247) (-17.4417, 45.0986) (-17.4725, 45.0741) (-17.5053, 45.0517) (-17.5394, 45.0311) (-17.5748, 45.0123) (-17.6115, 44.9956) (-17.6494, 44.9814) (-17.6883, 44.9691) (-17.7283, 44.9589) (-17.7694, 44.951) (-17.8115, 44.9457) (-17.8547, 44.9421) (-17.8838, 44.9418) (-17.8986, 44.9416) knots 0 0 0 0 0.061674 0.123053 0.183475 0.243727 0.304279 0.364863 0.425946 0.487391 0.54922 0.611144 0.673529 0.736961 0.800785 0.866013 0.932101 1 1 1 1
  spline S21 degree 3 poles (-17.8986, 44.9416) (-17.9126, 44.9417) (-17.9402, 44.9419) (-17.981, 44.945) (-18.0208, 44.9493) (-18.0593, 44.9557) (-18.0969, 44.9633) (-18.1331, 44.9734) (-18.1684, 44.9847) (-18.2026, 44.9981) (-18.2356, 45.0131) (-18.2675, 45.0301) (-18.2982, 45.0489) (-18.328, 45.0692) (-18.3565, 45.0914) (-18.3838, 45.1155) (-18.4102, 45.1411) (-18.4266, 45.1597) (-18.4348, 45.169) knots 0 0 0 0 0.069663 0.13775 0.203917 0.26878 0.332414 0.394754 0.45618 0.516996 0.577396 0.637198 0.696999 0.756756 0.816554 0.876948 0.938132 1 1 1 1
  spline S22 degree 3 poles (-18.4348, 45.169) (-18.448, 45.1851) (-18.4741, 45.2173) (-18.5076, 45.2694) (-18.5363, 45.3238) (-18.5594, 45.3808) (-18.5775, 45.4402) (-18.5901, 45.5022) (-18.5982, 45.5665) (-18.5992, 45.6103) (-18.5996, 45.6325) knots 0 0 0 0 0.124329 0.247156 0.36878 0.490734 0.613614 0.738958 0.867311 1 1 1 1
  line L47 (-15.527, 46.225) -> (-15.7398, 46.225)
  line L48 (-15.9273, 45.125) -> (-15.527, 46.225)
  line L49 (-15.4273, 45.125) -> (-15.9273, 45.125)
  line L50 (-15.027, 46.225) -> (-15.4273, 45.125)
  line L51 (-14.8141, 46.225) -> (-15.027, 46.225)
  line L52 (-15.2145, 45.125) -> (-14.8141, 46.225)
  line L53 (-15.0145, 45.125) -> (-15.2145, 45.125)
  line L54 (-15.0873, 44.925) -> (-15.0145, 45.125)
  line L55 (-16.213, 44.925) -> (-15.0873, 44.925)
  line L56 (-15.7398, 46.225) -> (-16.213, 44.925)
  line L57 (-20.903, 44.975) -> (-20.9196, 44.975)
  line L58 (-20.9196, 44.975) -> (-21.4696, 46.275)
  line L59 (-21.4696, 46.275) -> (-21.3446, 46.275)
  line L60 (-21.3446, 46.275) -> (-20.9113, 45.2505)
  line L61 (-20.9113, 45.2505) -> (-20.478, 46.275)
  line L62 (-20.478, 46.275) -> (-20.353, 46.275)
  line L63 (-20.353, 46.275) -> (-20.903, 44.975)
  spline S23 degree 3 poles (-21.713, 45.6244) (-21.7132, 45.6046) (-21.7137, 45.5658) (-21.7161, 45.5092) (-21.7209, 45.4557) (-21.727, 45.4052) (-21.7353, 45.3581) (-21.7456, 45.3139) (-21.7569, 45.2727) (-21.771, 45.2348) (-21.7864, 45.1995) (-21.8031, 45.1666) (-21.821, 45.1357) (-21.8406, 45.1071) (-21.8614, 45.0806) (-21.8839, 45.0566) (-21.9076, 45.0346) (-21.9326, 45.0151) (-21.9588, 44.998) (-21.9855, 44.9826) (-22.0133, 44.9703) (-22.0415, 44.9597) (-22.0705, 44.9516) (-22.1003, 44.946) (-22.1308, 44.9421) (-22.1513, 44.9418) (-22.1617, 44.9416) knots 0 0 0 0 0.065063 0.126773 0.185516 0.240765 0.29298 0.34225 0.388919 0.432776 0.474628 0.514775 0.553606 0.591426 0.628028 0.663804 0.698984 0.733591 0.767628 0.801208 0.834264 0.866981 0.89972 0.932702 0.966176 1 1 1 1
  spline S24 degree 3 poles (-22.1617, 44.9416) (-22.1719, 44.9418) (-22.1921, 44.9421) (-22.2221, 44.9457) (-22.2512, 44.9514) (-22.2795, 44.9593) (-22.3073, 44.9691) (-22.334, 44.9817) (-22.3601, 44.9963) (-22.3855, 45.013) (-22.4097, 45.032) (-22.4327, 45.0531) (-22.4541, 45.0768) (-22.4741, 45.1026) (-22.493, 45.1303) (-22.5104, 45.1604) (-22.5265, 45.1926) (-22.5412, 45.2273) (-22.5543, 45.2649) (-22.5658, 45.3058) (-22.5749, 45.3504) (-22.5827, 45.3983) (-22.589, 45.4499) (-22.5933, 45.5049) (-22.596, 45.5636) (-22.5962, 45.6038) (-22.5963, 45.6244) knots 0 0 0 0 0.033787 0.066622 0.099285 0.131361 0.163585 0.196104 0.228902 0.262158 0.295991 0.330218 0.36506 0.400951 0.43762 0.475708 0.515381 0.556414 0.599765 0.646424 0.696431 0.749782 0.806573 0.867436 0.931887 1 1 1 1
  spline S25 degree 3 poles (-22.5963, 45.6244) (-22.5962, 45.6453) (-22.5959, 45.6858) (-22.5933, 45.7447) (-22.5889, 45.8001) (-22.5829, 45.8517) (-22.5757, 45.8998) (-22.5659, 45.9441) (-22.5548, 45.9848) (-22.542, 46.0221) (-22.5275, 46.0565) (-22.5118, 46.0886) (-22.4941, 46.1184) (-22.4755, 46.1463) (-22.4553, 46.1719) (-22.434, 46.1955) (-22.4109, 46.2166) (-22.3866, 46.2359) (-22.3609, 46.2528) (-22.3347, 46.2677) (-22.3077, 46.2804) (-22.2798, 46.2903) (-22.2513, 46.2986) (-22.2221, 46.3042) (-22.1921, 46.3078) (-22.1719, 46.3081) (-22.1617, 46.3083) knots 0 0 0 0 0.068595 0.133246 0.194313 0.251279 0.304513 0.354235 0.400481 0.443411 0.484015 0.523252 0.561042 0.5979 0.633518 0.668314 0.702496 0.736685 0.770293 0.803437 0.835913 0.86846 0.900847 0.933467 0.966258 1 1 1 1
  spline S26 degree 3 poles (-22.1617, 46.3083) (-22.1513, 46.3081) (-22.1308, 46.3078) (-22.1004, 46.3043) (-22.0707, 46.2985) (-22.0418, 46.2904) (-22.0135, 46.2803) (-21.9861, 46.2676) (-21.9593, 46.2529) (-21.9335, 46.2356) (-21.9085, 46.2163) (-21.885, 46.1945) (-21.8628, 46.1703) (-21.8418, 46.1442) (-21.8224, 46.1155) (-21.804, 46.0847) (-21.7875, 46.0514) (-21.7717, 46.016) (-21.7579, 45.9777) (-21.7456, 45.9365) (-21.7356, 45.8921) (-21.7273, 45.8447) (-21.7209, 45.794) (-21.7162, 45.7402) (-21.7137, 45.6833) (-21.7132, 45.6444) (-21.713, 45.6244) knots 0 0 0 0 0.033788 0.067194 0.099862 0.132567 0.165151 0.197913 0.231319 0.265083 0.299255 0.334399 0.369943 0.406284 0.444064 0.482998 0.523354 0.565537 0.609613 0.656391 0.705885 0.758325 0.813832 0.872795 0.934722 1 1 1 1
  line L64 (-27.863, 45.625) -> (-27.7296, 46.275)
  line L65 (-27.7296, 46.275) -> (-27.1963, 46.275)
  line L66 (-27.1963, 46.275) -> (-27.1963, 46.1416)
  line L67 (-27.1963, 46.1416) -> (-27.6385, 46.1416)
  line L68 (-27.6385, 46.1416) -> (-27.7085, 45.7997)
  spline S27 degree 3 poles (-27.7085, 45.7997) (-27.6948, 45.8035) (-27.6681, 45.8109) (-27.6288, 45.819) (-27.5914, 45.824) (-27.5672, 45.8246) (-27.5554, 45.825) knots 0 0 0 0 0.275068 0.532901 0.773973 1 1 1 1
  spline S28 degree 3 poles (-27.5554, 45.825) (-27.5409, 45.8247) (-27.5124, 45.824) (-27.4706, 45.8181) (-27.4307, 45.8088) (-27.3928, 45.7957) (-27.3569, 45.779) (-27.3231, 45.7582) (-27.2911, 45.7339) (-27.2614, 45.7059) (-27.2345, 45.6751) (-27.2108, 45.642) (-27.1907, 45.6068) (-27.1745, 45.5694) (-27.1616, 45.5301) (-27.153, 45.4884) (-27.1473, 45.4447) (-27.1466, 45.4149) (-27.1463, 45.3997) knots 0 0 0 0 0.065808 0.129394 0.190894 0.251281 0.310815 0.370371 0.430768 0.492881 0.555104 0.616067 0.677256 0.73826 0.800762 0.864778 0.931045 1 1 1 1
  spline S29 degree 3 poles (-27.1463, 45.3997) (-27.1466, 45.3891) (-27.147, 45.3681) (-27.1495, 45.3368) (-27.1543, 45.3062) (-27.1608, 45.2763) (-27.1692, 45.2471) (-27.1793, 45.2185) (-27.1917, 45.1907) (-27.2053, 45.1635) (-27.2206, 45.1374) (-27.2376, 45.113) (-27.2556, 45.0899) (-27.2749, 45.0685) (-27.2958, 45.0487) (-27.318, 45.0305) (-27.3413, 45.0136) (-27.366, 44.9987) (-27.3917, 44.985) (-27.4187, 44.9737) (-27.4463, 44.9636) (-27.4751, 44.9556) (-27.5048, 44.9493) (-27.5356, 44.945) (-27.5673, 44.9419) (-27.5888, 44.9417) (-27.5997, 44.9416) knots 0 0 0 0 0.044014 0.087434 0.130118 0.172554 0.214555 0.256298 0.298438 0.340849 0.382715 0.423924 0.464246 0.504074 0.543862 0.583567 0.623094 0.663229 0.703551 0.743938 0.784541 0.82575 0.867757 0.910745 0.954914 1 1 1 1
  spline S30 degree 3 poles (-27.5997, 44.9416) (-27.6126, 44.9419) (-27.6381, 44.9424) (-27.6755, 44.9477) (-27.7114, 44.9552) (-27.7456, 44.9666) (-27.7784, 44.9809) (-27.8094, 44.9989) (-27.8394, 45.0193) (-27.867, 45.0434) (-27.8927, 45.0698) (-27.9157, 45.0983) (-27.9362, 45.1287) (-27.9538, 45.161) (-27.9689, 45.1951) (-27.9807, 45.2312) (-27.9902, 45.269) (-27.9943, 45.2951) (-27.9963, 45.3083) knots 0 0 0 0 0.065421 0.128708 0.190236 0.250724 0.310637 0.370766 0.431615 0.493523 0.555883 0.617342 0.678668 0.740711 0.802985 0.866803 0.932347 1 1 1 1
  line L69 (-27.9963, 45.3083) -> (-27.8796, 45.3083)
  spline S31 degree 3 poles (-27.8796, 45.3083) (-27.8768, 45.2959) (-27.8713, 45.2721) (-27.8591, 45.2386) (-27.8443, 45.2088) (-27.8267, 45.1822) (-27.8057, 45.159) (-27.7818, 45.1383) (-27.7549, 45.1197) (-27.725, 45.1042) (-27.6935, 45.0909) (-27.6606, 45.0821) (-27.627, 45.0759) (-27.6043, 45.0753) (-27.5929, 45.075) knots 0 0 0 0 0.094687 0.181994 0.264377 0.34218 0.418618 0.496509 0.577369 0.661511 0.746733 0.831258 0.915206 1 1 1 1
  spline S32 degree 3 poles (-27.5929, 45.075) (-27.5818, 45.0753) (-27.5599, 45.0759) (-27.5276, 45.0805) (-27.4965, 45.0876) (-27.4668, 45.0983) (-27.438, 45.1112) (-27.4108, 45.1278) (-27.3845, 45.1469) (-27.3598, 45.1688) (-27.3372, 45.1929) (-27.3172, 45.2188) (-27.3006, 45.2463) (-27.2866, 45.2751) (-27.276, 45.3054) (-27.2684, 45.3372) (-27.2639, 45.3704) (-27.2633, 45.3931) (-27.263, 45.4047) knots 0 0 0 0 0.064207 0.126425 0.18768 0.248216 0.308305 0.369661 0.431699 0.495947 0.559758 0.622295 0.683911 0.745092 0.80674 0.869087 0.93329 1 1 1 1
  spline S33 degree 3 poles (-27.263, 45.4047) (-27.2632, 45.4151) (-27.2637, 45.4355) (-27.2676, 45.4654) (-27.2744, 45.4936) (-27.2839, 45.5204) (-27.2958, 45.5457) (-27.3105, 45.5697) (-27.3281, 45.5918) (-27.3482, 45.6123) (-27.3702, 45.6312) (-27.3945, 45.6473) (-27.4206, 45.6608) (-27.4482, 45.6725) (-27.4779, 45.6809) (-27.5091, 45.6872) (-27.5422, 45.6909) (-27.5649, 45.6914) (-27.5765, 45.6916) knots 0 0 0 0 0.065351 0.127916 0.18836 0.247216 0.30563 0.36377 0.422661 0.482687 0.5433 0.604118 0.664965 0.727413 0.791468 0.858055 0.927037 1 1 1 1
  spline S34 degree 3 poles (-27.5765, 45.6916) (-27.5866, 45.6914) (-27.6074, 45.691) (-27.6393, 45.6877) (-27.6728, 45.6824) (-27.7079, 45.6751) (-27.7445, 45.6656) (-27.7827, 45.6542) (-27.8224, 45.6406) (-27.8492, 45.6303) (-27.863, 45.625) knots 0 0 0 0 0.102203 0.211023 0.3251 0.446502 0.573788 0.708901 0.850358 1 1 1 1
  line L70 (0, 0) -> (-7.5, 0)
  circle A17 centre (0, 0) radius 7.5 projected
  line L71 (-11.163, -50.525) -> (-11.6756, -50.525)
  line L72 (-11.6756, -50.525) -> (-11.7673, -49.091)
  arc A18 (-11.7673, -49.091) -> (-15.9587, -49.091) centre (-13.863, -49.225) ccw
  line L73 (-15.9587, -49.091) -> (-16.0504, -50.525)
  line L74 (-16.0504, -50.525) -> (-20.3387, -50.525)
  arc A19 (-20.4094, -50.4957) -> (-20.3387, -50.525) centre (-20.3387, -50.425) ccw
  line L75 (-20.4094, -50.4957) -> (-20.7337, -50.1714)
  arc A20 (-20.7337, -50.1714) -> (-21.0872, -50.025) centre (-21.0872, -50.525) ccw
  line L76 (-21.0872, -50.025) -> (-30.763, -50.025)
  arc A21 (-30.863, -49.925) -> (-30.763, -50.025) centre (-30.763, -49.925) ccw
  line L77 (-30.863, -49.925) -> (-30.863, -40.775)
  arc A22 (-30.763, -40.675) -> (-30.863, -40.775) centre (-30.763, -40.775) ccw
  line L78 (-30.763, -40.675) -> (-27.8372, -40.675)
  arc A23 (-27.8372, -40.675) -> (-27.4837, -40.5285) centre (-27.8372, -40.175) ccw
  line L79 (-27.4837, -40.5285) -> (-27.1594, -40.2043)
  arc A24 (-27.0887, -40.175) -> (-27.1594, -40.2043) centre (-27.0887, -40.275) ccw
  line L80 (-27.0887, -40.175) -> (-24.3372, -40.175)
  arc A25 (-24.2665, -40.2043) -> (-24.3372, -40.175) centre (-24.3372, -40.275) ccw
  line L81 (-24.2665, -40.2043) -> (-23.9423, -40.5285)
  arc A26 (-23.9423, -40.5285) -> (-23.5887, -40.675) centre (-23.5887, -40.175) ccw
  line L82 (-23.5887, -40.675) -> (-18.3372, -40.675)
  arc A27 (-18.3372, -40.675) -> (-17.9837, -40.5285) centre (-18.3372, -40.175) ccw
  line L83 (-17.9837, -40.5285) -> (-17.6594, -40.2043)
  arc A28 (-17.5887, -40.175) -> (-17.6594, -40.2043) centre (-17.5887, -40.275) ccw
  line L84 (-17.5887, -40.175) -> (-14.8372, -40.175)
  arc A29 (-14.7665, -40.2043) -> (-14.8372, -40.175) centre (-14.8372, -40.275) ccw
  line L85 (-14.7665, -40.2043) -> (-14.4423, -40.5285)
  arc A30 (-14.4423, -40.5285) -> (-14.0887, -40.675) centre (-14.0887, -40.175) ccw
  line L86 (-14.0887, -40.675) -> (-11.163, -40.675)
  arc A31 (-11.063, -40.775) -> (-11.163, -40.675) centre (-11.163, -40.775) ccw
  line L87 (-11.063, -40.775) -> (-11.063, -50.425)
  arc A32 (-11.163, -50.525) -> (-11.063, -50.425) centre (-11.163, -50.425) ccw
  circle A33 centre (-16.213, -42.725) radius 1.25
  circle A34 centre (-25.713, -42.725) radius 1.25
  line L88 (-26.8863, -44.975) -> (-26.2696, -46.275)
  line L89 (-26.2696, -46.275) -> (-26.253, -46.275)
  line L90 (-26.253, -46.275) -> (-25.653, -44.975)
  line L91 (-25.653, -44.975) -> (-25.7798, -44.975)
  line L92 (-25.7798, -44.975) -> (-25.972, -45.3916)
  line L93 (-25.972, -45.3916) -> (-26.5613, -45.3916)
  line L94 (-26.5613, -45.3916) -> (-26.759, -44.975)
  line L95 (-26.759, -44.975) -> (-26.8863, -44.975)
  spline S35 degree 3 poles (-24.0663, -45.9114) (-24.0665, -45.9203) (-24.067, -45.9378) (-24.0711, -45.9634) (-24.0773, -45.9881) (-24.0862, -46.012) (-24.098, -46.0348) (-24.1122, -46.0566) (-24.1287, -46.0777) (-24.1478, -46.0974) (-24.1688, -46.1155) (-24.1909, -46.1315) (-24.2143, -46.1449) (-24.2389, -46.1559) (-24.2646, -46.1645) (-24.2915, -46.1705) (-24.3195, -46.1742) (-24.3386, -46.1747) (-24.3483, -46.175) knots 0 0 0 0 0.061965 0.122122 0.180988 0.239933 0.299906 0.359989 0.421776 0.486576 0.551535 0.615018 0.677259 0.73973 0.80305 0.866495 0.931973 1 1 1 1
  spline S36 degree 3 poles (-24.3483, -46.175) (-24.3585, -46.1747) (-24.3785, -46.1742) (-24.4078, -46.1705) (-24.4357, -46.1642) (-24.4624, -46.1556) (-24.4879, -46.1447) (-24.512, -46.1311) (-24.5347, -46.1148) (-24.556, -46.0964) (-24.5756, -46.0758) (-24.5929, -46.0529) (-24.6079, -46.0281) (-24.6211, -46.0014) (-24.6318, -45.9726) (-24.6399, -45.9418) (-24.6464, -45.9091) (-24.6485, -45.8865) (-24.6496, -45.875) knots 0 0 0 0 0.064439 0.126547 0.186887 0.245878 0.304041 0.362191 0.420976 0.48066 0.5406 0.600689 0.661936 0.724443 0.789038 0.856314 0.926352 1 1 1 1
  line L96 (-24.6496, -45.875) -> (-24.7663, -45.875)